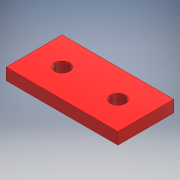
# Autodesk Inventor part: soportes celda de carga
Saved by Autodesk Inventor 2018 (Build 220112000, 112)
## iProperties
Created: 2019-05-18
Part Number: soportes celda de carga
Material: Generic
Document SubType Name: Modeling
Designer: JLVega003
Density: 1 g/cm^3
Appearance: Light Red
Author: JLVega003
Autodesk Inventor part; units mm, degrees
ref_plane "YZ Plane" through (0, 0, 0) normal (1, 0, 0) x (0, 1, 0)
ref_plane "XZ Plane" through (0, 0, 0) normal (0, 1, 0) x (-1, 0, 0)
ref_plane "XY Plane" through (0, 0, 0) normal (0, 0, 1) x (1, 0, 0)
sketch "Sketch1" plane through (0, 0, 0) normal (0, 0, 1) x (1, 0, 0)
  line L0 (15, -7.5) -> (-15, -7.5)
  line L1 (-15, -7.5) -> (-15, 7.5)
  line L2 (-15, 7.5) -> (15, 7.5)
  line L3 (15, 7.5) -> (15, -7.5)
  line L4 (15, -7.5) -> (-15, 7.5) construction
  line L5 (-15, -7.5) -> (15, 7.5) construction
  circle A0 centre (-7.5, 0) radius 2
  circle A1 centre (7.5, 0) radius 2
  line L6 (-21, 0) -> (21, 0) projected
  line L7 (0, -10.5) -> (0, 10.5) projected
  line L8 (-7.5, 0) -> (7.5, 0)
  point P0 (0, 0)
  point P1 (0, 0)
  dimension "d10" = 30
  dimension "d11" = 15
  dimension "d12" = 4
  dimension "d13" = 15
  constraints: 14 end point, 4 midpoint, 2 centre point, 2 parallel, 1 collinear, 1 equal radius, 1 horizontal, 1 perpendicular
  measures "d10" distance between parallel lines of L3 L1
  measures "d11" distance of L8.end L8.start
  measures "d12" diameter of A1
  measures "d13" distance between parallel lines of L0 L2
extrude "Extrusion1" add sketch "Sketch1" along normal blind 3.175 contours L0 L7 L6 A1 L3 | L0 L1 L6 A0 L7 | L6 A1 L7 L2 L3 | L6 A0 L1 L2 L7
body "Solid1"
